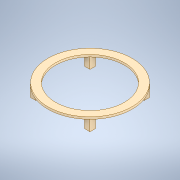
# Autodesk Inventor part: Tarcza_Podkładka
Saved by Autodesk Inventor 2022 (Build 260153000, 153)
## iProperties
Created: 2021-06-13
Part Number: Tarcza_Podkładka
Material: Polietylen o dużej gęstości
Document SubType Name: Modeling
Designer: Matik
Density: 0.952 g/cm^3
Appearance: Gładki — w kolorze złamanej bieli
Author: Matik
Autodesk Inventor part; units mm, degrees
ref_plane "YZ Plane" through (0, 0, 0) normal (1, 0, 0) x (0, 1, 0)
ref_plane "XZ Plane" through (0, 0, 0) normal (0, 1, 0) x (-1, 0, 0)
ref_plane "XY Plane" through (0, 0, 0) normal (0, 0, 1) x (1, 0, 0)
sketch "Szkic1" plane through (0, 0, 0) normal (0, 1, 0) x (-1, 0, 0)
  line L0 (-25, -25) -> (25, -25)
  line L1 (25, -25) -> (25, 25)
  line L2 (25, 25) -> (-25, 25)
  line L3 (-25, 25) -> (-25, -25)
  line L4 (-25, -25) -> (25, 25) construction
  line L5 (25, -25) -> (-25, 25) construction
  line L6 (22.5, 22.5) -> (27.5, 22.5)
  line L7 (27.5, 22.5) -> (27.5, 27.5)
  line L8 (27.5, 27.5) -> (22.5, 27.5)
  line L9 (22.5, 27.5) -> (22.5, 22.5)
  line L10 (22.5, 22.5) -> (27.5, 27.5) construction
  line L11 (27.5, 22.5) -> (22.5, 27.5) construction
  line L12 (27.5, -27.5) -> (22.5, -27.5)
  line L13 (22.5, -27.5) -> (22.5, -22.5)
  line L14 (22.5, -22.5) -> (27.5, -22.5)
  line L15 (27.5, -22.5) -> (27.5, -27.5)
  line L16 (27.5, -27.5) -> (22.5, -22.5) construction
  line L17 (22.5, -27.5) -> (27.5, -22.5) construction
  line L18 (-27.5, -22.5) -> (-22.5, -22.5)
  line L19 (-22.5, -22.5) -> (-22.5, -27.5)
  line L20 (-22.5, -27.5) -> (-27.5, -27.5)
  line L21 (-27.5, -27.5) -> (-27.5, -22.5)
  line L22 (-27.5, -22.5) -> (-22.5, -27.5) construction
  line L23 (-22.5, -22.5) -> (-27.5, -27.5) construction
  line L24 (-27.5, 27.5) -> (-22.5, 27.5)
  line L25 (-22.5, 27.5) -> (-22.5, 22.5)
  line L26 (-22.5, 22.5) -> (-27.5, 22.5)
  line L27 (-27.5, 22.5) -> (-27.5, 27.5)
  line L28 (-27.5, 27.5) -> (-22.5, 22.5) construction
  line L29 (-22.5, 27.5) -> (-27.5, 22.5) construction
  circle A0 centre (0, 0) radius 35.3553
  circle A1 centre (0, 0) radius 38.8909
  circle A2 centre (0, 0) radius 31.8198
  point P0 (-19.685, 25)
  point P1 (19.685, 25)
  point P2 (25, 19.685)
  point P3 (25, -19.685)
  point P4 (19.685, -25)
  point P5 (-19.685, -25)
  point P6 (-25, -19.685)
  point P7 (-25, 19.685)
  dimension "d14" = 63.6396
  dimension "d0" = 50
  dimension "d1" = 50
  dimension "d2" = 5
  dimension "d3" = 5
  dimension "d4" = 5
  dimension "d5" = 5
  dimension "d6" = 5
  dimension "d7" = 5
  dimension "d8" = 5
  dimension "d9" = 5
  constraints: 60 end point, 10 midpoint, 10 parallel, 5 horizontal, 5 perpendicular, 2 coincident, 9 other
  measures "d0" distance of L2.end L1.end
  measures "d1" distance of L1.end L0.end
  measures "d2" distance of L8.end L7.end
  measures "d3" distance of L7.end L6.end
  measures "d4" distance of L13.end L14.end
  measures "d5" distance of L12.end L13.end
  measures "d6" distance of L19.end L20.end
  measures "d7" distance of L18.start L20.end
  measures "d8" distance of L25.end L26.end
  measures "d9" distance of L24.end L25.end
extrude "Wyciągnięcie proste1" add sketch "Szkic1" along normal blind 2 contours L3 L18 L19 L0 | A0 L18 L3 | A0 L19 L20 L21 L18 | L0 L19 A0 | L19 A2 L0 | L0 A2 L13 A0 L19 | L18 A0 L26 L3 A2 | L3 A2 L18 | L18 L21 A1 L27 L26 A0 | A0 L13 L12 A1 L20 L19 | A0 L3 L26 | L26 L27 L24 L25 A0 | A0 L14 L15 L12 L13 | L13 L0 A0 | A2 L13 L0 | L3 L26 A2 | L3 L2 L25 L26 | A0 L25 L2 | L13 L14 L1 L0 | L1 L14 A0 | A2 L1 L14 | L25 L2 A2 | A1 L8 L9 A0 L25 L24 | L15 L14 A0 L6 L7 A1 | L25 A0 L9 L2 A2 | L1 A2 L6 A0 L14 | L7 L6 A0 L9 L8 | A0 L2 L9 | A2 L6 L1 | L2 L9 A2 | L2 L1 L6 L9 | A0 L6 L1
extrude "Wyciągnięcie proste2" add sketch "Szkic1" against normal blind 10 contours L3 L18 L19 L0 | A0 L18 L3 | A0 L19 L20 L21 L18 | L0 L19 A0 | A0 L3 L26 | L26 L27 L24 L25 A0 | A0 L14 L15 L12 L13 | L13 L0 A0 | L3 L2 L25 L26 | A0 L25 L2 | L13 L14 L1 L0 | L1 L14 A0 | L7 L6 A0 L9 L8 | A0 L2 L9 | L2 L1 L6 L9 | A0 L6 L1
equation "\"d7\" = d6"
